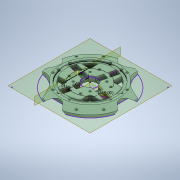
# Autodesk Inventor part: bord_mount
Saved by Autodesk Inventor 2020 (Build 240168000, 168)
## iProperties
Created: 2024-09-13
Part Number: bord_mount
Material: Типовые
Document SubType Name: Modeling
Designer: Ivan
Density: 1 g/cm^3
Appearance: Резина — зеленая
Author: Ivan
Autodesk Inventor part; units mm, degrees
ref_plane "YZ Plane" through (0, 0, 0) normal (1, 0, 0) x (0, 1, 0)
ref_plane "XY Plane" through (0, 0, 0) normal (0, 0, 1) x (1, 0, 0)
sketch "Эскиз1" plane through (0, 0, 0) normal (0, 1, 0) x (-1, 0, 0)
  arc A0 (-31, 99.2724) -> (-99.2724, 31) centre (0, 0) ccw
  arc A1 (31, -99.2724) -> (99.2724, -31) centre (0, 0) ccw
  arc A2 (-34.57, -98.0863) -> (-98.0863, -34.57) centre (-109.0212, -109.0212) ccw
  arc A3 (34.57, 98.0863) -> (98.0863, 34.57) centre (109.0212, 109.0212) ccw
  arc A4 (-34.57, -98.0863) -> (-31, -99.2724) centre (0, 0) ccw
  arc A5 (-99.2724, -31) -> (-98.0863, -34.57) centre (0, 0) ccw
  line L0 (-99.2724, 31) -> (-78.7724, 31)
  line L1 (-78.7724, 31) -> (-78.7724, -31)
  line L2 (-78.7724, -31) -> (-99.2724, -31)
  line L3 (-31, 99.2724) -> (-31, 78.7724)
  line L4 (-31, 78.7724) -> (31, 78.7724)
  line L5 (31, 78.7724) -> (31, 99.2724)
  line L6 (99.2724, 31) -> (78.7724, 31)
  line L7 (78.7724, 31) -> (78.7724, -31)
  line L8 (78.7724, -31) -> (99.2724, -31)
  line L9 (-31, -99.2724) -> (-31, -78.7724)
  line L10 (-31, -78.7724) -> (31, -78.7724)
  line L11 (31, -78.7724) -> (31, -99.2724)
  circle A6 centre (-42.22, 16) radius 1.5
  circle A7 centre (-72.43, 16) radius 1.5
  circle A8 centre (-42.22, -16) radius 1.5
  circle A9 centre (-72.43, -16) radius 1.5
  circle A10 centre (-72.43, -31) radius 1.5
  circle A11 centre (-16, -42.22) radius 1.5
  circle A12 centre (-31, -72.43) radius 1.5
  circle A13 centre (-16, -72.43) radius 1.5
  circle A14 centre (16, -72.43) radius 1.5
  circle A15 centre (44.87, -82.9015) radius 1.5
  circle A16 centre (57.67, -74.5664) radius 1.5
  circle A17 centre (16, -42.22) radius 1.5
  circle A18 centre (74.5664, -57.67) radius 1.5
  circle A19 centre (82.9015, -44.87) radius 1.5
  circle A20 centre (42.22, -16) radius 1.5
  circle A21 centre (72.43, -16) radius 1.5
  circle A22 centre (72.43, 16) radius 1.5
  circle A23 centre (42.22, 16) radius 1.5
  circle A24 centre (72.43, 31) radius 1.5
  circle A25 centre (31, 72.43) radius 1.5
  circle A26 centre (16, 72.43) radius 1.5
  circle A27 centre (16, 42.22) radius 1.5
  circle A28 centre (-16, 42.22) radius 1.5
  circle A29 centre (-16, 72.43) radius 1.5
  circle A30 centre (-44.87, 82.9015) radius 1.5
  circle A31 centre (-57.67, 74.5664) radius 1.5
  circle A32 centre (-74.5664, 57.67) radius 1.5
  circle A33 centre (-82.9015, 44.87) radius 1.5
  line L12 (-73.5391, 73.5391) -> (73.5391, -73.5391) construction
  arc A34 (99.2724, 31) -> (98.0863, 34.57) centre (0, 0) ccw
  arc A35 (34.57, 98.0863) -> (31, 99.2724) centre (0, 0) ccw
  arc A36 (-98.0863, -34.57) -> (-34.57, -98.0863) centre (0, 0) ccw
  arc A37 (98.0863, 34.57) -> (34.57, 98.0863) centre (0, 0) ccw
  constraints: 38 centre point, 26 end point, 23 point on circle, 5 coincident, 1 horizontal, 1 perpendicular, 1 symmetric about line, 2 other
sketch "Эскиз2" plane through (0, 0, 0) normal (0, 1, 0) x (-1, 0, 0)
  line L0 (22, 49.72) -> (-22, 49.72) construction
  line L1 (-22, 49.72) -> (-22, 34.72) construction
  line L2 (-22, 34.72) -> (22, 34.72) construction
  line L3 (22, 34.72) -> (22, 49.72) construction
  line L4 (-22, 42.22) -> (22, 42.22) construction
  line L5 (0, 49.72) -> (0, 34.72) construction
  circle A0 centre (16, 42.22) radius 1.5 construction
  line L6 (-34.72, 22) -> (-49.72, 22) construction
  line L7 (-49.72, 22) -> (-49.72, -22) construction
  line L8 (-34.72, -22) -> (-34.72, 22) construction
  line L9 (-49.72, -22) -> (-34.72, -22) construction
  line L10 (-22, -34.72) -> (-22, -49.72) construction
  line L11 (-22, -49.72) -> (22, -49.72) construction
  line L12 (22, -34.72) -> (-22, -34.72) construction
  line L13 (22, -49.72) -> (22, -34.72) construction
  line L14 (34.72, -22) -> (49.72, -22) construction
  line L15 (49.72, -22) -> (49.72, 22) construction
  line L16 (34.72, 22) -> (34.72, -22) construction
  line L17 (49.72, 22) -> (34.72, 22) construction
  circle A1 centre (0, 0) radius 104
  arc A2 (-34.57, -98.0863) -> (-98.0863, -34.57) centre (-109.0212, -109.0212) ccw construction
  arc A3 (34.57, 98.0863) -> (98.0863, 34.57) centre (109.0212, 109.0212) ccw construction
  point P0 (-42.22, 22)
  point P1 (-49.72, 0)
  point P2 (-34.72, 0)
  point P3 (-42.22, -22)
  point P4 (-22, -42.22)
  point P5 (0, -49.72)
  point P6 (0, -34.72)
  point P7 (22, -42.22)
  point P8 (42.22, -22)
  point P9 (49.72, 0)
  point P10 (34.72, 0)
  point P11 (42.22, 22)
  point P12 (31, -99.2724)
  dimension "d0" = 15
  dimension "d1" = 44
  dimension "d4" = 360
  constraints: 36 end point, 5 point on circle, 4 midpoint, 3 centre point, 3 coincident, 2 parallel, 2 point on line, 1 horizontal, 1 perpendicular, 49 other
  measures "d0" distance of L2.end L0.start
  measures "d1" distance of L0.end L0.start
sketch "Эскиз3" plane through (0, 0, 0) normal (1, 0, 0) x (0, 1, 0)
  line L0 (0, -104) -> (0, 104) construction
  line L1 (0, 104) -> (0, 0)
  line L2 (0, 104) -> (7, 104)
  line L3 (7, 104) -> (7, 78.7724)
  line L4 (7, 78.7724) -> (0, 78.7724)
  line L5 (0, 78.7724) -> (0, 104)
  line L6 (15, 80.7724) -> (7, 104)
  line L7 (7, 78.7724) -> (0, 78.7724)
  line L8 (0, 78.7724) -> (0, 65.7724)
  line L9 (0, 65.7724) -> (7, 65.7724)
  line L10 (7, 65.7724) -> (7, 78.7724)
  line L11 (15, 80.7724) -> (15, 73.2724)
  line L12 (15, 73.2724) -> (12, 73.2724)
  line L13 (12, 73.2724) -> (12, 65.7724)
  line L14 (12, 65.7724) -> (7, 65.7724)
  line L15 (-3, 0) -> (18, 0) projected
  line L16 (15, 80.7724) -> (7, 80.7724)
  dimension "d6" = 7
  dimension "d8" = 13
  dimension "d130" = 7.5
  dimension "d131" = 15
  dimension "d133" = 3
  dimension "d134" = 5
  constraints: 30 end point, 6 perpendicular, 4 parallel, 2 horizontal, 2 point on line, 2 vertical
  measures "d6" distance of L3.end L4.end
  measures "d8" distance of L8.end L7.end
  measures "d130" distance of L12.end L13.end
  measures "d131" distance from line of L14 L16.end
  measures "d133" distance of L11.end L12.end
  measures "d134" distance of L13.end L9.end
revolve "Вращение1" add sketch "Эскиз3" angle 360 about axis through (0, 0, 0) along (0, 1, 0)
hole "Отверстие1" at (16, 0, 72.43) at (-16, 0, 72.43) at (72.43, 0, 16) at (72.43, 0, -16) at (16, 0, -72.43) at (-16, 0, -72.43) at (-72.43, 0, -16) at (-72.43, 0, 16) at (-72.43, 0, 31) at (-31, 0, 72.43) at (72.43, 0, -31) at (31, 0, -72.43) direction (0, 1, 0) diameter 3.3 end through all
ref_plane "РабПлоскость1" through (0, 4, 0) normal (0, -1, 0) x (1, 0, 0)
ref_plane "РабПлоскость2" through (-34.72, 0, 22) normal (-1, 0, 0) x (0, 0, -1)
sketch "Эскиз6" plane through (-34.72, 0, 22) normal (-1, 0, 0) x (0, 0, -1)
  line L0 (22, 35.7857) -> (22, -23.4643) projected
  line L1 (53, -14) -> (-9, -14)
  line L2 (-9, -14) -> (-9, 0)
  line L3 (-9, 0) -> (53, 0)
  line L4 (53, 0) -> (53, -14)
  line L5 (-82, 0) -> (126, 0) construction
  arc A0 (-9, 0) -> (53, 0) centre (22, 27.3214) ccw
  point P0 (22, 0)
  point P1 (22, -14)
  dimension "d64" = 62
  dimension "d65" = 14
  constraints: 8 end point, 2 midpoint, 2 parallel, 2 point on circle, 1 centre point, 1 horizontal, 1 perpendicular, 1 point on line
  measures "d64" distance of L2.end L3.end
  measures "d65" distance of L1.end L2.end
extrude "Выдавливание2" cut sketch "Эскиз6" along normal blind 100 and the other way blind 200 contours L3 A0 L0 | L0 A0 L3
pattern_circular "Круговой массив1" count 2 over 90 about axis through (0, 0, 0) along (0, 1, 0) of "Выдавливание2"
ref_plane "РабПлоскость3" through (-0.3641, 0, -1) normal (0, -1, 0) x (1, 0, 0)
extrude "Выдавливание6" cut sketch "Эскиз1" along normal through all contours A37 A3 | A2 A36
extrude "Выдавливание7" add sketch "Эскиз6" along normal up to surface (44.0524 mm away) contours L3 A0 L0 | L0 A0 L3
pattern_circular "Круговой массив2" count 4 over 360 about axis through (0, 0, 0) along (0, 1, 0) of "Выдавливание7"
extrude "Выдавливание8" add sketch "Эскиз6" along normal up to surface contours A0 L4 L1 | L1 L2 A0 round surface about axis through (0, 6, 0) along (0, 1, 0) radius 65.7724 far side no
pattern_circular "Круговой массив3" count 4 over 360 about axis through (0, 0, 0) along (0, 1, 0) of "Выдавливание8"
sketch "Эскиз9" plane through (-99.2724, 0, 31) normal (0, -1, 0) x (1, 0, 0)
  line L0 (133.9924, -62) -> (133.9924, 0) projected
  circle A0 centre (99.2724, -31) radius 46.5454
  circle A1 centre (99.2724, -31) radius 20
  dimension "d78" = 40
  constraints: 2 coincident, 1 centre point, 3 other
  measures "d78" diameter of A1
extrude "Выдавливание9" add sketch "Эскиз9" against normal up to surface (14 mm away) contours A0 L0 picked at (129.0857, -31)
sketch "Эскиз10" plane through (0, 14, 0) normal (0, 1, 0) x (0.9700415, 0, 0.2429394)
  line L0 (8, -18.3303) -> (-8, -18.3303)
  line L1 (-8, -18.3303) -> (-8, -65.284)
  line L2 (-8, -65.284) -> (8, -65.284)
  line L3 (8, -65.284) -> (8, -18.3303)
  line L4 (-8, -65.284) -> (8, -18.3303) construction
  arc A0 (-59.516, -27.9974) -> (-48.7397, -44.1639) centre (0, 0) ccw construction
  line L5 (0, -65.7724) -> (0, 65.7724) construction
  circle A1 centre (0, 0) radius 20 construction
  line L6 (18.3303, -8) -> (65.284, -8)
  line L7 (65.284, -8) -> (65.284, 8)
  line L8 (65.284, 8) -> (18.3303, 8)
  line L9 (18.3303, 8) -> (18.3303, -8)
  line L10 (8, 18.3303) -> (8, 65.284)
  line L11 (8, 65.284) -> (-8, 65.284)
  line L12 (-8, 65.284) -> (-8, 18.3303)
  line L13 (-8, 18.3303) -> (8, 18.3303)
  line L14 (-18.3303, 8) -> (-65.284, 8)
  line L15 (-65.284, 8) -> (-65.284, -8)
  line L16 (-65.284, -8) -> (-18.3303, -8)
  line L17 (-18.3303, -8) -> (-18.3303, 8)
  point P0 (0, 0)
  point P1 (0, -41.8072)
  dimension "d79" = 16
  dimension "d82" = 360
  constraints: 36 end point, 3 point on circle, 2 midpoint, 2 parallel, 1 horizontal, 1 perpendicular, 1 point on line, 1 vertical, 35 other
  measures "d79" distance of L0.start L0.end
extrude "Выдавливание10" cut sketch "Эскиз10" against normal blind 10.9
ref_plane "РабПлоскость4" through (0, 11.5, 0) normal (0, 1, 0) x (0.9700415, 0, 0.2429394)
sketch "Эскиз11" plane through (0, 11.5, 0) normal (0, 1, 0) x (0.9700415, 0, 0.2429394)
  line L0 (-8, -65.284) -> (-8, -18.3303) projected
  line L1 (-8, -46.8072) -> (8, -46.8072)
  line L2 (8, -46.8072) -> (8, -36.8072)
  line L3 (8, -36.8072) -> (-8, -36.8072)
  line L4 (-8, -36.8072) -> (-8, -46.8072)
  line L5 (-8, -65.284) -> (-8, -18.3303) projected
  line L6 (46.8072, -8) -> (46.8072, 8)
  line L7 (36.8072, -8) -> (46.8072, -8)
  line L8 (36.8072, 8) -> (36.8072, -8)
  line L9 (46.8072, 8) -> (36.8072, 8)
  line L10 (8, 46.8072) -> (-8, 46.8072)
  line L11 (8, 36.8072) -> (8, 46.8072)
  line L12 (-8, 36.8072) -> (8, 36.8072)
  line L13 (-8, 46.8072) -> (-8, 36.8072)
  line L14 (-46.8072, 8) -> (-46.8072, -8)
  line L15 (-36.8072, 8) -> (-46.8072, 8)
  line L16 (-36.8072, -8) -> (-36.8072, 8)
  line L17 (-46.8072, -8) -> (-36.8072, -8)
  line L18 (8, -18.3303) -> (8, -65.284) projected
  point P0 (0, 0)
  point P1 (-8, -41.8072)
  point P2 (41.8072, -8)
  point P3 (8, 41.8072)
  point P4 (-41.8072, 8)
  point P5 (-8, -36.8072)
  dimension "d87" = 10
  dimension "d90" = 360
  constraints: 32 end point, 2 midpoint, 2 parallel, 2 point on line, 1 horizontal, 1 perpendicular, 37 other
  measures "d87" distance of L3.end L1.start
extrude "Выдавливание11" add sketch "Эскиз11" along normal up to surface (2.5 mm away)
sketch "Эскиз5" plane through (0, 4, 0) normal (0, -1, 0) x (1, 0, 0)
  arc A0 (71.8308, 14.4626) -> (71.239, 17.1419) centre (72.43, 16) ccw projected
  arc A1 (71.239, -17.1419) -> (71.8308, -14.4626) centre (72.43, -16) ccw projected
  arc A2 (14.4626, -71.8308) -> (17.1419, -71.239) centre (16, -72.43) ccw projected
  arc A3 (-17.1419, -71.239) -> (-14.4626, -71.8308) centre (-16, -72.43) ccw projected
  arc A4 (-71.8308, -14.4626) -> (-71.239, -17.1419) centre (-72.43, -16) ccw projected
  arc A5 (-71.239, 17.1419) -> (-71.8308, 14.4626) centre (-72.43, 16) ccw projected
  arc A6 (-14.4626, 71.8308) -> (-17.1419, 71.239) centre (-16, 72.43) ccw projected
  arc A7 (17.1419, 71.239) -> (14.4626, 71.8308) centre (16, 72.43) ccw projected
  circle A8 centre (-31, 72.43) radius 1.65 projected
  circle A9 centre (16, 72.43) radius 3
  circle A10 centre (-16, 72.43) radius 3
  circle A11 centre (-31, 72.43) radius 3
  circle A12 centre (-72.4023, 30.9882) radius 1.6497
  circle A13 centre (-72.4023, 30.9882) radius 3
  circle A14 centre (-72.43, 16) radius 3
  circle A15 centre (-72.43, -16) radius 1.65 projected
  circle A16 centre (-72.43, -16) radius 3
  circle A17 centre (-16, -72.43) radius 1.65 projected
  circle A18 centre (-16, -72.43) radius 3
  circle A19 centre (16, -72.43) radius 3
  circle A20 centre (72.43, -16) radius 1.65 projected
  circle A21 centre (72.43, -16) radius 3
  circle A22 centre (72.43, 16) radius 3
  circle A23 centre (31, -72.43) radius 1.65 projected
  line L0 (31, -70.78) -> (31.005, -74.08) construction
  circle A24 centre (31, -72.43) radius 1.65 projected
  circle A25 centre (31, -72.43) radius 3
  circle A26 centre (72.43, -31) radius 1.65 projected
  line L1 (72.43, -29.35) -> (72.3791, -32.6492) construction
  circle A27 centre (72.43, -31) radius 1.65 projected
  circle A28 centre (72.43, -31) radius 3
  point P0 (0, 0)
  point P1 (-32.5048, 71.7532)
  point P2 (-29.4715, 73.0514)
  dimension "d18" = 6
  dimension "d19" = 6
  dimension "d20" = 6
  dimension "d21" = 6
  dimension "d22" = 6
  dimension "d23" = 6
  dimension "d24" = 6
  dimension "d25" = 6
  dimension "d26" = 6
  dimension "d27" = 6
  dimension "d28" = 6
  dimension "d29" = 6
  constraints: 13 centre point, 12 coincident, 6 point on circle, 4 end point, 5 other
  measures "d18" diameter of A9
  measures "d19" diameter of A10
  measures "d20" diameter of A11
  measures "d21" diameter of A13
  measures "d22" diameter of A14
  measures "d23" diameter of A16
  measures "d24" diameter of A18
  measures "d25" diameter of A19
  measures "d26" diameter of A21
  measures "d27" diameter of A22
  measures "d28" diameter of A25
  measures "d29" diameter of A28
extrude "Выдавливание1" cut sketch "Эскиз5" against normal through all contours A20 A1 | A17 A3 | A15 A4 | A8 | A9 | A10 | A11 | A12 | A13 | A14 | A16 | A18 | A19 | A21 | A22 | A23 | A25 | A26 | A28
sketch "Эскиз12" plane through (0, 12, 0) normal (0, 1, 0) x (1, 0, 0)
  arc A0 (-31, -58.0086) -> (-8, -65.284) centre (0, 0) ccw projected
  line L0 (-8, -65.284) -> (8, -65.284)
  line L1 (-3.611, -47.3484) -> (-1.1816, -37.648) projected
  arc A1 (-13.0175, -72.1067) -> (13.0175, -72.1067) centre (0, 0) ccw projected
  line L2 (-23.6204, -61.3847) -> (-19.1316, -43.4614) projected
  line L3 (-8, -65.284) -> (-8, -72.8343)
  line L4 (8, -65.284) -> (8, -72.8343)
  line L5 (65.284, -8) -> (72.8343, -8)
  line L6 (65.284, -8) -> (65.284, 8)
  line L7 (65.284, 8) -> (72.8343, 8)
  line L8 (8, 65.284) -> (8, 72.8343)
  line L9 (8, 65.284) -> (-8, 65.284)
  line L10 (-8, 65.284) -> (-8, 72.8343)
  line L11 (-65.284, 8) -> (-72.8343, 8)
  line L12 (-65.284, 8) -> (-65.284, -8)
  line L13 (-65.284, -8) -> (-72.8343, -8)
  arc A2 (-72.1067, 13.0175) -> (-72.1067, -13.0175) centre (0, 0) ccw projected
  arc A3 (13.0175, 72.1067) -> (-13.0175, 72.1067) centre (0, 0) ccw projected
  arc A4 (72.1067, -13.0175) -> (72.1067, 13.0175) centre (0, 0) ccw projected
  point P0 (-3.611, -47.3484)
  point P1 (-19.1316, -43.4614)
  point P2 (-1.1816, -37.648)
  dimension "d96" = 360
  constraints: 24 end point, 2 point on circle, 1 parallel, 1 vertical, 31 other
extrude "Выдавливание12" cut sketch "Эскиз12" against normal up to surface (8.9 mm away)
extrude "Выдавливание13" cut sketch "Эскиз1" along normal blind 10.9 contours A10 | A12 | A24 | A25
sketch "Эскиз13" plane through (0, 15, 0) normal (0, 1, 0) x (0.7071068, 0, 0.7071068)
  circle A0 centre (39.902, -62.5295) radius 3 projected
  circle A1 centre (62.5295, -39.902) radius 3 projected
  circle A2 centre (-39.902, -62.5295) radius 3 projected
  circle A3 centre (-62.5295, -39.902) radius 3 projected
  circle A4 centre (-62.5295, 39.902) radius 3 projected
  circle A5 centre (-39.902, 62.5295) radius 3 projected
  circle A6 centre (39.902, 62.5295) radius 3 projected
  circle A7 centre (62.5295, 39.902) radius 3 projected
  circle A8 centre (90.3481, -26.8923) radius 3
  circle A9 centre (90.3481, 26.8923) radius 3
  circle A10 centre (-90.3481, -26.8923) radius 3
  circle A11 centre (-90.3481, 26.8923) radius 3
  circle A12 centre (41.1678, -18.5403) radius 3
  circle A13 centre (41.1678, 18.5403) radius 3
  circle A14 centre (18.5403, 41.1678) radius 3
  circle A15 centre (-18.5403, 41.1678) radius 3
  circle A16 centre (-41.1678, 18.5403) radius 3
  circle A17 centre (-41.1678, -18.5403) radius 3
  circle A18 centre (-18.5403, -41.1678) radius 3
  circle A19 centre (18.5403, -41.1678) radius 3
  point P0 (0, 0)
  dimension "d102" = 6
  dimension "d103" = 6
  dimension "d104" = 6
  dimension "d105" = 6
  dimension "d106" = 6
  dimension "d107" = 6
  dimension "d108" = 6
  dimension "d109" = 6
  dimension "d110" = 6
  dimension "d111" = 6
  dimension "d112" = 6
  dimension "d113" = 6
  constraints: 12 centre point, 12 coincident
  measures "d102" diameter of A8
  measures "d103" diameter of A9
  measures "d104" diameter of A10
  measures "d105" diameter of A11
  measures "d106" diameter of A12
  measures "d107" diameter of A13
  measures "d108" diameter of A14
  measures "d109" diameter of A15
  measures "d110" diameter of A16
  measures "d111" diameter of A17
  measures "d112" diameter of A18
  measures "d113" diameter of A19
extrude "Выдавливание14" cut sketch "Эскиз13" against normal through all
sketch "Эскиз14" plane through (65.284, 12, 8) normal (0, 1, 0) x (1, 0, 0)
  arc A0 (5.5964, -10.5688) -> (6.8227, -5.0175) centre (7.146, -8) ccw projected
  circle A1 centre (-65.284, 8) radius 73.2724
  line L0 (-3.8993, -15.6204) -> (-21.8226, -11.1316) projected
  line L1 (-21.8226, 0) -> (7.5503, 0)
  arc A2 (6.8227, -5.0175) -> (6.8227, 21.0175) centre (-65.284, 8) ccw projected
  line L2 (-17.9356, 4.389) -> (-21.8226, -11.1316) projected
  line L3 (-45.5593, 11.3072) -> (-0.0123, -0.0997) projected
  line L4 (-17.9356, 16) -> (7.5503, 16)
  line L5 (-73.284, 54.8072) -> (-73.284, 80.8343)
  line L6 (-57.284, 54.8072) -> (-57.284, 80.8343)
  line L7 (-112.0912, 0) -> (-138.1183, 0)
  line L8 (-112.0912, 16) -> (-138.1183, 16)
  line L9 (-57.284, -38.8072) -> (-57.284, -64.8343)
  line L10 (-73.284, -38.8072) -> (-73.284, -64.8343)
  circle A3 centre (-65.284, 8) radius 20
  point P0 (0, 0)
  point P1 (7.5503, 0)
  point P2 (-45.5593, 11.3072)
  point P3 (-0.0123, -0.0997)
  dimension "d118" = 360
  constraints: 16 end point, 2 centre point, 2 coincident, 2 horizontal, 2 point on circle, 27 other
sketch "Эскиз15" plane through (-58.0086, 14, -31) normal (0, 1, 0) x (1, 0, 0)
  circle A0 centre (58.0086, -31) radius 20
  circle A1 centre (58.0086, -31) radius 33.25 construction
  line L0 (58.0086, -31) -> (81.5199, -7.4887) construction
  line L1 (58.0086, -31) -> (91.2586, -31) construction
  circle A2 centre (81.5199, -7.4887) radius 2.8
  circle A3 centre (34.4973, -7.4887) radius 2.8
  circle A4 centre (34.4973, -54.5113) radius 2.8
  circle A5 centre (81.5199, -54.5113) radius 2.8
  point P0 (58.0086, -31)
  dimension "d123" = 66.5
  dimension "d122" = 40
  dimension "d124" = 45
  dimension "d125" = 5.6
  dimension "d126" = 360
  constraints: 5 centre point, 4 end point, 3 coincident, 1 equal length, 1 horizontal, 12 other
  measures "d122" diameter of A0
  measures "d124" angle of L1 L0
  measures "d125" diameter of A2
extrude "Выдавливание15" cut sketch "Эскиз15" against normal blind 9.2 contours A2 | A3 | A4 | A5
equation "\"d130\" = 0.5 * d131"
equation "\"d19\" = d18"
equation "\"d20\" = d18"
equation "\"d21\" = d18"
equation "\"d22\" = d18"
equation "\"d23\" = d18"
equation "\"d24\" = d18"
equation "\"d25\" = d18"
equation "\"d26\" = d18"
equation "\"d27\" = d18"
equation "\"d28\" = d18"
equation "\"d29\" = d18"
